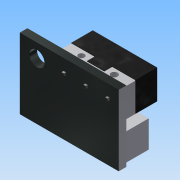
# Autodesk Inventor part: концевик
Saved by Autodesk Inventor 2017 (Build 210142000, 142)
## iProperties
Part Number: концевик
Material: Типовые
Document SubType Name: Modeling
Designer: chucha
Density: 1 g/cm^3
Appearance: Оружейный металл — полированный
Mass: 0.936935 g
Surface Area: 11.9295 cm^2
Volume: 0.936935 cm^3
Author: chucha
Autodesk Inventor part; units mm, degrees
ref_plane "YZ Plane" through (0, 0, 0) normal (1, 0, 0) x (0, 1, 0)
ref_plane "XZ Plane" through (0, 0, 0) normal (0, 1, 0) x (-1, 0, 0)
sketch "Эскиз1" plane through (0, 0, 0) normal (0, 0, 1) x (1, 0, 0)
  line L0 (0, 0) -> (0, 34.3761) construction
  line L1 (0, 0) -> (-29.3608, 0) construction
  circle A0 centre (-10, 0) radius 1.65
  circle A1 centre (-10, 0) radius 3.45
  circle A2 centre (10, 0) radius 1.65
  circle A3 centre (10, 0) radius 3.45
  line L2 (-10, 3.45) -> (10, 3.45)
  line L3 (-6.5, -3.45) -> (-6.5, -9.66)
  line L4 (-6.5, -9.66) -> (6.5, -9.66)
  line L5 (6.5, -9.66) -> (6.5, -3.45)
  line L6 (-10, -3.45) -> (-6.5, -3.45)
  line L7 (6.5, -3.45) -> (10, -3.45)
  line L8 (-4.98, -7.06) -> (4.98, -7.06)
  line L9 (4.98, -7.06) -> (4.98, -14)
  line L10 (4.98, -14) -> (-4.98, -14)
  line L11 (-4.98, -14) -> (-4.98, -7.06)
  line L12 (-6.38, 8.03) -> (6.38, 8.03)
  line L13 (-6.38, 3.7894) -> (-1.7, 3.7894)
  line L14 (-1.7, 3.7894) -> (-1.7, 2.21)
  line L15 (-1.7, 2.21) -> (1.7, 2.21)
  line L16 (1.7, 2.21) -> (1.7, 3.7894)
  line L17 (1.7, 3.7894) -> (6.38, 3.7894)
  line L18 (-6.38, 3.6894) -> (-6.29, 3.6894)
  line L19 (-6.29, 3.6894) -> (-6.29, 3.7894)
  line L20 (6.38, 3.6894) -> (6.29, 3.6894)
  line L21 (6.29, 3.6894) -> (6.29, 3.7894)
  line L22 (-6.38, 1.91) -> (-6.38, 3.6894)
  line L23 (-6.38, 3.7894) -> (-6.38, 8.03)
  line L24 (6.38, 8.03) -> (6.38, 3.7894)
  line L25 (6.38, 3.6894) -> (6.38, 1.91)
  line L26 (-6.38, 1.91) -> (-4.4028, 1.91)
  line L27 (-4.4028, 1.91) -> (-4, 1.43)
  line L28 (6.38, 1.91) -> (4.4028, 1.91)
  line L29 (4.4028, 1.91) -> (4, 1.43)
  line L30 (-2.5, 1.43) -> (-2.0972, 1.91)
  line L31 (-2.0972, 1.91) -> (2.0972, 1.91)
  line L32 (2.0972, 1.91) -> (2.5, 1.43)
  circle A4 centre (-3.25, 2.6493) radius 0.6032
  circle A5 centre (3.25, 2.6493) radius 0.6676
  line L33 (-3.25, 2.6493) -> (-3.25, 0.6364) construction
  line L34 (3.25, 2.6493) -> (3.25, 0.375) construction
  line L35 (4, 1.43) -> (2.5, 1.43)
  line L36 (-2.5, 1.43) -> (-4, 1.43)
  circle A6 centre (10, 0) radius 3.45
  dimension "d0" = 3.3
  dimension "d1" = 6.9
  dimension "d2" = 3.3
  dimension "d3" = 6.9
  dimension "d4" = 20
  dimension "d5" = 26.9
  dimension "d6" = 13.11
  dimension "d7" = 6.21
  dimension "d8" = 13
  dimension "d9" = 2.6
  dimension "d10" = 6.94
  dimension "d11" = 9.96
  dimension "d14" = 4.58
  dimension "d15" = 0.1
  dimension "d16" = 6.38
  dimension "d17" = 6.38
  dimension "d18" = 6.38
  dimension "d19" = 6.38
  dimension "d20" = 6.12
  dimension "d21" = 0.3
  dimension "d22" = 6.6
  dimension "d23" = 130
  dimension "d24" = 3.4
  dimension "d25" = 6.5
  dimension "d26" = 1.5
  constraints: 74 end point, 14 parallel, 10 perpendicular, 7 horizontal, 6 centre point, 5 point on line, 4 collinear, 4 point on circle, 4 vertical, 3 coincident, 3 tangent, 2 symmetric about line, 1 vertical alignment, 9 other
  measures "d0" diameter of A0
  measures "d1" diameter of A1
  measures "d2" diameter of A2
  measures "d3" diameter of A3
  measures "d4" distance of A0.centre A2.centre
  measures "d6" distance between parallel lines of L2 L4
  measures "d7" distance between parallel lines of L4 L6
  measures "d8" distance between parallel lines of L5 L3
  measures "d9" distance between parallel lines of L4 L8
  measures "d10" distance between parallel lines of L10 L8
  measures "d11" distance between parallel lines of L9 L11
  measures "d14" distance between parallel lines of L12 L2
  measures "d15" distance between parallel lines of L18 L13
  measures "d16" distance between parallel lines of L0 L23
  measures "d17" distance between parallel lines of L0 L24
  measures "d18" distance between parallel lines of L0 L22
  measures "d19" distance between parallel lines of L0 L25
  measures "d20" distance between parallel lines of L12 L26
  measures "d21" distance between parallel lines of L31 L15
  measures "d22" distance between parallel lines of L12 L36
  measures "d23" angle of L26 L27
  measures "d24" distance between parallel lines of L16 L14
  measures "d25" distance between parallel lines of L34 L33
  measures "d26" distance of L30.start L27.end
extrude "Выдавливание1" add sketch "Эскиз1" against normal blind 1.55 contours A1 | A1 L2 L22 L26 L27 L36 L30 L31 L32 L35 L29 L28 L25 A3 L7 L5 L4 L9 L8 L11 L3 L6 | L2 L14 L15 L16 L25 L28 L29 L35 L32 L31 L30 L36 L27 L26 L22 | L2 L16 L15 L14 | L11 L8 L9 L4 | A3 | A4 | A5
extrude "Выдавливание2" add sketch "Эскиз1" along normal blind 5.8 contours L14 L13 L23 L12 L24 L17 L16 L2 | L2 L16 L15 L14
extrude "Выдавливание3" add sketch "Эскиз1" along normal blind 5.7 contours L22 L18 L19 L13 L14 L2 | L2 L14 L15 L16 L25 L28 L29 L35 L32 L31 L30 L36 L27 L26 L22 | L16 L17 L21 L20 L25 L2
extrude "Выдавливание4" add sketch "Эскиз1" along normal blind 0.05 contours A1 | A3
extrude "Выдавливание5" add sketch "Эскиз1" along normal blind 5.8 contours L11 L8 L9 L4 | L4 L9 L10 L11
sketch "Эскиз2" plane through (-4.98, -14, 0) normal (0, -1, 0) x (1, 0, 0)
  line L0 (9.96, 0) -> (0, 0) projected
  line L1 (9.96, 0) -> (9.96, 5.8) projected
  line L2 (0, 5.8) -> (9.96, 5.8) projected
  line L3 (0, 0) -> (0, 5.8) projected
  line L4 (4.98, 0) -> (4.98, 10.0399) construction
  line L5 (0, 0) -> (0, 5.8) construction
  line L6 (0, 2.9) -> (8.4494, 2.9) construction
  line L7 (9.41, 0.55) -> (0.55, 0.55)
  line L8 (0.55, 0.55) -> (0.55, 5.25)
  line L9 (0.55, 5.25) -> (9.41, 5.25)
  line L10 (9.41, 5.25) -> (9.41, 0.55)
  line L11 (9.41, 0.55) -> (0.55, 5.25) construction
  line L12 (0.55, 0.55) -> (9.41, 5.25) construction
  line L13 (0, 5.25) -> (9.96, 5.25)
  line L14 (9.96, 5.25) -> (9.96, 4.05)
  line L15 (9.96, 4.05) -> (0, 4.05)
  line L16 (0, 4.05) -> (0, 5.25)
  line L17 (9.96, 5.8) -> (0, 5.8) projected
  line L18 (1.78, 5.25) -> (3.58, 5.25)
  line L19 (3.58, 5.25) -> (3.58, 5.8)
  line L20 (3.58, 5.8) -> (1.78, 5.8)
  line L21 (1.78, 5.8) -> (1.78, 5.25)
  line L22 (6.38, 5.25) -> (8.18, 5.25)
  line L23 (8.18, 5.25) -> (8.18, 5.8)
  line L24 (8.18, 5.8) -> (6.38, 5.8)
  line L25 (6.38, 5.8) -> (6.38, 5.25)
  line L26 (-3.9038, 3.4362) -> (13.6375, 3.4362) construction
  line L27 (5.23, 3.6862) -> (4.73, 3.6862)
  line L28 (4.73, 3.6862) -> (4.73, 3.1862)
  line L29 (4.73, 3.1862) -> (5.23, 3.1862)
  line L30 (5.23, 3.1862) -> (5.23, 3.6862)
  line L31 (5.23, 3.6862) -> (4.73, 3.1862) construction
  line L32 (4.73, 3.6862) -> (5.23, 3.1862) construction
  line L33 (2.73, 3.6862) -> (2.23, 3.6862)
  line L34 (2.23, 3.6862) -> (2.23, 3.1862)
  line L35 (2.23, 3.1862) -> (2.73, 3.1862)
  line L36 (2.73, 3.1862) -> (2.73, 3.6862)
  line L37 (2.73, 3.6862) -> (2.23, 3.1862) construction
  line L38 (2.23, 3.6862) -> (2.73, 3.1862) construction
  line L39 (7.23, 3.6862) -> (7.73, 3.6862)
  line L40 (7.73, 3.6862) -> (7.73, 3.1862)
  line L41 (7.73, 3.1862) -> (7.23, 3.1862)
  line L42 (7.23, 3.1862) -> (7.23, 3.6862)
  line L43 (7.23, 3.6862) -> (7.73, 3.1862) construction
  line L44 (7.73, 3.6862) -> (7.23, 3.1862) construction
  line L45 (0.5772, 0) -> (0.5772, 5.7) projected
  line L46 (0, 5.25) -> (0.5772, 5.25)
  line L47 (0.5772, 5.25) -> (0.5772, 4.05)
  line L48 (0.5772, 4.05) -> (0, 4.05)
  line L49 (0, 4.05) -> (0, 5.25)
  line L50 (9.96, 5.25) -> (9.41, 5.25)
  line L51 (9.41, 5.25) -> (9.41, 4.05)
  line L52 (9.41, 4.05) -> (9.96, 4.05)
  line L53 (9.96, 4.05) -> (9.96, 5.25)
  line L54 (8.18, 5.25) -> (6.38, 5.25)
  line L55 (6.38, 5.25) -> (6.38, 5.8)
  line L56 (6.38, 5.8) -> (8.18, 5.8)
  line L57 (8.18, 5.8) -> (8.18, 5.25)
  line L58 (3.58, 5.25) -> (1.78, 5.25)
  line L59 (1.78, 5.25) -> (1.78, 5.8)
  line L60 (1.78, 5.8) -> (3.58, 5.8)
  line L61 (3.58, 5.8) -> (3.58, 5.25)
  point P0 (4.98, 2.9)
  point P1 (4.98, 3.4362)
  point P2 (2.48, 3.4362)
  point P3 (7.48, 3.4362)
  dimension "d37" = 0.55
  dimension "d38" = 0.55
  dimension "d39" = 1.2
  dimension "d40" = 1.8
  dimension "d41" = 1.8
  dimension "d42" = 2.8
  dimension "d43" = 0.5
  dimension "d44" = 0.5
  dimension "d45" = 0.5
  dimension "d46" = 0.5
  dimension "d47" = 5
  constraints: 110 end point, 22 parallel, 18 point on line, 13 horizontal, 11 perpendicular, 9 midpoint, 1 collinear, 1 symmetric about line, 1 vertical, 1 other
  measures "d37" distance between parallel lines of L2 L9
  measures "d38" distance between parallel lines of L3 L8
  measures "d39" distance between parallel lines of L15 L13
  measures "d40" distance between parallel lines of L23 L25
  measures "d41" distance between parallel lines of L21 L19
  measures "d42" distance between parallel lines of L25 L19
  measures "d43" distance of L29.end L28.end
  measures "d44" distance of L28.end L27.end
  measures "d45" distance of L35.end L34.end
  measures "d46" distance of L40.end L41.end
  measures "d47" distance of point (2.48, 3.436) point (7.48, 3.436)
extrude "Выдавливание6" cut sketch "Эскиз2" against normal blind 5.3 contours L45 L15 L10 L7 | L7 L8 L15 L45 | L15 L45 L9 L10 | L15 L8 L9 L45
extrude "Выдавливание7" cut sketch "Эскиз2" against normal blind 3.2 contours L15 L10 L13 L1 | L3 L13 L8 L15 | L15 L8 L9 L45 | L23 L9 L25 L2 | L21 L2 L19 L9
sketch "Эскиз3" plane through (0, 0, 0) normal (1, 0, 0) x (0, 1, 0)
  line L0 (2.5743, 3.55) -> (-0.5, 3.55)
  line L1 (0, 3.05) -> (2.5743, 3.05)
  line L2 (2.5743, 3.05) -> (2.5743, 3.55)
  line L3 (0, 3.05) -> (0, 0)
  line L4 (0, 0) -> (-0.5, 0)
  line L5 (-0.5, 0) -> (-0.5, 3.55)
  line L6 (-7.06, 0) -> (-7.06, 5.8) projected
  line L7 (-3.45, 0) -> (-9.66, 0) projected
  line L8 (-7.06, 3.686) -> (-6.36, 3.686)
  line L9 (-6.36, 3.686) -> (-6.36, 0)
  line L10 (-6.36, 0) -> (-7.06, 0)
  line L11 (-7.06, 0) -> (-7.06, 3.686)
  line L12 (-7.06, 3.186) -> (-6.86, 3.186)
  line L13 (-6.86, 3.186) -> (-6.86, 0)
  line L14 (-6.86, 0) -> (-7.06, 0)
  line L15 (-7.06, 0) -> (-7.06, 3.186)
  line L16 (1.91, 0) -> (1.91, 5.7) projected
  line L17 (3.45, 0.05) -> (-3.45, 0.05) projected
  dimension "d52" = 3.686
  dimension "d53" = 0.5
  dimension "d54" = 0.5
  dimension "d55" = 0.2
  dimension "d56" = 0.5
  dimension "d57" = 0.5
  dimension "d58" = 2.41
  dimension "d59" = 3.5
  constraints: 28 end point, 6 parallel, 4 point on line, 3 horizontal, 2 perpendicular
  measures "d52" distance between parallel lines of L7 L8
  measures "d53" distance between parallel lines of L8 L12
  measures "d54" distance between parallel lines of L9 L13
  measures "d55" distance between parallel lines of L6 L13
  measures "d56" distance between parallel lines of L5 L3
  measures "d57" distance between parallel lines of L0 L1
  measures "d58" distance between parallel lines of L16 L5
  measures "d59" distance between parallel lines of L17 L0
extrude "Выдавливание9" add sketch "Эскиз3" along normal mid plane 0.5 contours L2 L1 L16 L0 | L16 L1 L3 L17 L5 L0 | L17 L3 L4 L5
pattern_linear "Прямоуг.массив1" count 3 spacing 4.32 along (1, 0, 0) of "Выдавливание9" first direction both ways yes
extrude "Выдавливание10" add sketch "Эскиз3" along normal mid plane 0.5 contours L6 L8 L9 L7 L13 L12
pattern_linear "Прямоуг.массив2" count 3 spacing 1.9 along (1, 0, 0) of "Выдавливание10" first direction both ways yes
sketch "Эскиз4" plane through (0, 0, -1.55) normal (0, 0, -1) x (-1, 0, 0)
  line L0 (-1.65, -6.86) -> (-1.65, -6.36) projected
  line L1 (-1.65, -6.36) -> (-2.15, -6.36) projected
  line L2 (-2.15, -6.36) -> (-2.15, -6.86) projected
  line L3 (-2.15, -6.86) -> (-1.65, -6.86) projected
  line L4 (2.15, -6.86) -> (2.15, -6.36) projected
  line L5 (2.15, -6.36) -> (1.65, -6.36) projected
  line L6 (1.65, -6.36) -> (1.65, -6.86) projected
  line L7 (1.65, -6.86) -> (2.15, -6.86) projected
  line L8 (0.25, -6.86) -> (0.25, -6.36) projected
  line L9 (0.25, -6.36) -> (-0.25, -6.36) projected
  line L10 (-0.25, -6.36) -> (-0.25, -6.86) projected
  line L11 (-0.25, -6.86) -> (0.25, -6.86) projected
  line L12 (-4.07, -0.5) -> (-4.07, 0) projected
  line L13 (-4.07, 0) -> (-4.57, 0) projected
  line L14 (-4.57, 0) -> (-4.57, -0.5) projected
  line L15 (-4.57, -0.5) -> (-4.07, -0.5) projected
  line L16 (4.57, -0.5) -> (4.57, 0) projected
  line L17 (4.57, 0) -> (4.07, 0) projected
  line L18 (4.07, 0) -> (4.07, -0.5) projected
  line L19 (4.07, -0.5) -> (4.57, -0.5) projected
  line L20 (0.25, -0.5) -> (0.25, 0) projected
  line L21 (0.25, 0) -> (-0.25, 0) projected
  line L22 (-0.25, 0) -> (-0.25, -0.5) projected
  line L23 (-0.25, -0.5) -> (0.25, -0.5) projected
  line L24 (-4.98, -7.06) -> (-4.98, -9.66) projected
  line L25 (-4.98, -9.66) -> (-6.5, -9.66) projected
  line L26 (-6.5, -9.66) -> (-6.5, -3.45) projected
  line L27 (-6.5, -3.45) -> (-10, -3.45) projected
  arc A0 (-10, -3.45) -> (-10, 3.45) centre (-10, 0) ccw projected
  line L28 (-10, 3.45) -> (-6.38, 3.45) projected
  line L29 (-6.38, 3.45) -> (-6.38, 1.91) projected
  line L30 (-6.38, 1.91) -> (-4.4028, 1.91) projected
  line L31 (-4.4028, 1.91) -> (-4, 1.43) projected
  line L32 (-4, 1.43) -> (-2.5, 1.43) projected
  line L33 (-2.5, 1.43) -> (-2.0972, 1.91) projected
  line L34 (-2.0972, 1.91) -> (2.0972, 1.91) projected
  line L35 (2.0972, 1.91) -> (2.5, 1.43) projected
  line L36 (2.5, 1.43) -> (4, 1.43) projected
  line L37 (4, 1.43) -> (4.4028, 1.91) projected
  line L38 (4.4028, 1.91) -> (6.38, 1.91) projected
  line L39 (6.38, 1.91) -> (6.38, 3.45) projected
  line L40 (6.38, 3.45) -> (10, 3.45) projected
  arc A1 (10, 3.45) -> (10, -3.45) centre (10, 0) ccw projected
  line L41 (10, -3.45) -> (6.5, -3.45) projected
  line L42 (6.5, -3.45) -> (6.5, -9.66) projected
  line L43 (6.5, -9.66) -> (4.98, -9.66) projected
  line L44 (4.98, -9.66) -> (4.98, -7.06) projected
  line L45 (4.98, -7.06) -> (-4.98, -7.06) projected
  point P0 (0, 0)
extrude "Выдавливание11" add sketch "Эскиз4" along normal blind 1.35 contours L3 L2 L1 L0 | L7 L6 L5 L4 | L11 L10 L9 L8 | L15 L14 L13 L12 | L19 L18 L17 L16 | L23 L22 L21 L20
fillet "Сопряжение1" radius 1.1 12 edges at (-1.9, -6.36, -1.55) (0, -6.36, -1.55) (1.9, -6.36, -1.55) (1.9, -6.86, -1.55) (0, -6.86, -1.55) (-1.9, -6.86, -1.55) (-4.32, -0.5, -1.55) (0, -0.5, -1.55) (4.32, -0.5, -1.55) (4.32, 0, -1.55) (0, 0, -1.55) (-4.32, 0, -1.55)
fillet "Сопряжение2" radius 0.6 12 edges at (-4.07, -0.25, -1.55) (0.25, -0.25, -1.55) (4.57, -0.25, -1.55) (2.15, -6.61, -1.55) (0.25, -6.61, -1.55) (-1.65, -6.61, -1.55) (1.65, -6.61, -1.55) (-0.25, -6.61, -1.55) (-2.15, -6.61, -1.55) (-4.57, -0.25, -1.55) (-0.25, -0.25, -1.55) (4.07, -0.25, -1.55)
sketch "Эскиз5" plane through (0, 0, -1.55) normal (0, 0, -1) x (-1, 0, 0)
  arc A0 (-10, -3.45) -> (-10, 3.45) centre (-10, 0) ccw projected
  arc A1 (10, 3.45) -> (10, -3.45) centre (10, 0) ccw projected
  circle A2 centre (-10, 0) radius 3.45
  line L0 (10, 3.45) -> (-10, 3.45) projected
  circle A3 centre (10, 0) radius 3.45
  point P0 (0, 0)
  constraints: 2 coincident, 2 vertical alignment, 4 other
extrude "Выдавливание12" cut sketch "Эскиз5" against normal blind 0.01
sketch "Эскиз6" plane through (0, 0, 0) normal (0, 0, 1) x (1, 0, 0)
  line L0 (-6.5, -3.45) -> (-6.5, -9.66) projected
  line L1 (6.5, -9.66) -> (6.5, -3.45) projected
  line L2 (-6.5, -3.45) -> (6.5, -3.45)
  line L3 (6.5, -3.45) -> (6.5, -4.7506)
  line L4 (6.5, -4.7506) -> (-6.5, -4.7506)
  line L5 (-6.5, -4.7506) -> (-6.5, -3.45)
  line L6 (-6.3, -3.65) -> (-3.3, -3.65)
  line L7 (-3.3, -3.65) -> (-3.3, -4.5506)
  line L8 (-3.3, -4.5506) -> (-6.3, -4.5506)
  line L9 (-6.3, -4.5506) -> (-6.3, -3.65)
  line L10 (3.3, -3.65) -> (6.3, -3.65)
  line L11 (6.3, -3.65) -> (6.3, -4.5506)
  line L12 (6.3, -4.5506) -> (3.3, -4.5506)
  line L13 (3.3, -4.5506) -> (3.3, -3.65)
  line L14 (0, 0) -> (0, -22.5011) construction
  line L15 (-3.1, -3.65) -> (-0.1, -3.65)
  line L16 (-0.1, -3.65) -> (-0.1, -4.5506)
  line L17 (-0.1, -4.5506) -> (-3.1, -4.5506)
  line L18 (-3.1, -4.5506) -> (-3.1, -3.65)
  line L19 (0.1, -3.65) -> (3.1, -3.65)
  line L20 (3.1, -3.65) -> (3.1, -4.5506)
  line L21 (3.1, -4.5506) -> (0.1, -4.5506)
  line L22 (0.1, -4.5506) -> (0.1, -3.65)
  line L23 (-6.1, -3.85) -> (-3.5, -3.85)
  line L24 (-3.5, -3.85) -> (-3.5, -4.3506)
  line L25 (-3.5, -4.3506) -> (-6.1, -4.3506)
  line L26 (-6.1, -4.3506) -> (-6.1, -3.85)
  line L27 (-2.9, -3.85) -> (-0.3, -3.85)
  line L28 (-0.3, -3.85) -> (-0.3, -4.3506)
  line L29 (-0.3, -4.3506) -> (-2.9, -4.3506)
  line L30 (-2.9, -4.3506) -> (-2.9, -3.85)
  line L31 (0.3, -3.85) -> (2.9, -3.85)
  line L32 (2.9, -3.85) -> (2.9, -4.3506)
  line L33 (2.9, -4.3506) -> (0.3, -4.3506)
  line L34 (0.3, -4.3506) -> (0.3, -3.85)
  line L35 (3.5, -3.85) -> (6.1, -3.85)
  line L36 (6.1, -3.85) -> (6.1, -4.3506)
  line L37 (6.1, -4.3506) -> (3.5, -4.3506)
  line L38 (3.5, -4.3506) -> (3.5, -3.85)
  line L39 (-5.6, -3.85) -> (-4, -3.85)
  line L40 (-4, -3.85) -> (-4, -4.3506)
  line L41 (-4, -4.3506) -> (-5.6, -4.3506)
  line L42 (-5.6, -4.3506) -> (-5.6, -3.85)
  line L43 (-2.4, -3.85) -> (-0.8, -3.85)
  line L44 (-0.8, -3.85) -> (-0.8, -4.3506)
  line L45 (-0.8, -4.3506) -> (-2.4, -4.3506)
  line L46 (-2.4, -4.3506) -> (-2.4, -3.85)
  line L47 (0.8, -3.85) -> (2.4, -3.85)
  line L48 (2.4, -3.85) -> (2.4, -4.3506)
  line L49 (2.4, -4.3506) -> (0.8, -4.3506)
  line L50 (0.8, -4.3506) -> (0.8, -3.85)
  line L51 (4, -3.85) -> (5.6, -3.85)
  line L52 (5.6, -3.85) -> (5.6, -4.3506)
  line L53 (5.6, -4.3506) -> (4, -4.3506)
  line L54 (4, -4.3506) -> (4, -3.85)
  dimension "d78" = 0.2
  dimension "d79" = 0.2
  dimension "d80" = 0.2
  dimension "d81" = 0.2
  dimension "d82" = 0.2
  dimension "d83" = 0.2
  dimension "d84" = 0.2
  dimension "d85" = 3
  dimension "d86" = 3
  dimension "d87" = 0.2
  dimension "d88" = 0.2
  dimension "d89" = 0.2
  dimension "d90" = 0.2
  dimension "d91" = 0.2
  dimension "d92" = 0.2
  dimension "d93" = 2.6
  dimension "d94" = 0.5
  dimension "d95" = 0.5
  dimension "d96" = 0.5
  dimension "d97" = 0.5
  constraints: 106 end point, 26 parallel, 19 point on line, 13 horizontal, 13 perpendicular, 2 collinear, 1 vertical, 11 other
  measures "d78" distance between parallel lines of L2 L6
  measures "d79" distance between parallel lines of L0 L9
  measures "d80" distance between parallel lines of L4 L8
  measures "d81" distance between parallel lines of L18 L7
  measures "d82" distance between parallel lines of L13 L20
  measures "d83" distance between parallel lines of L22 L16
  measures "d84" distance between parallel lines of L4 L17
  measures "d85" distance between parallel lines of L7 L9
  measures "d86" distance between parallel lines of L16 L18
  measures "d87" distance between parallel lines of L9 L26
  measures "d88" distance between parallel lines of L7 L24
  measures "d89" distance between parallel lines of L30 L18
  measures "d90" distance between parallel lines of L16 L28
  measures "d91" distance between parallel lines of L17 L29
  measures "d92" distance between parallel lines of L19 L31
  measures "d93" distance between parallel lines of L36 L38
  measures "d94" distance between parallel lines of L36 L52
  measures "d95" distance between parallel lines of L38 L54
  measures "d96" distance between parallel lines of L32 L48
  measures "d97" distance between parallel lines of L50 L34
extrude "Выдавливание13" add sketch "Эскиз6" along normal blind 0.01 contours L2 L1 L4 L0
extrude "Выдавливание14" add sketch "Эскиз6" along normal blind 0.8 contours L23 L40 L25 L42 | L27 L44 L29 L46 | L31 L48 L33 L50 | L35 L52 L37 L54
extrude "Выдавливание15" add sketch "Эскиз6" along normal blind 0.4 contours L23 L42 L25 L26 | L23 L40 L25 L42 | L23 L24 L25 L40 | L27 L46 L29 L30 | L27 L44 L29 L46 | L27 L28 L29 L44 | L31 L50 L33 L34 | L31 L48 L33 L50 | L31 L32 L33 L48 | L35 L54 L37 L38 | L35 L52 L37 L54 | L35 L36 L37 L52
fillet "Сопряжение3" radius 0.3 8 edges at (-5.6, -4.1003, 0.4) (-2.4, -4.1003, 0.4) (0.8, -4.1003, 0.4) (4, -4.1003, 0.4) (5.6, -4.1003, 0.4) (2.4, -4.1003, 0.4) (-0.8, -4.1003, 0.4) (-4, -4.1003, 0.4)
ref_plane "РабПлоскость1" through (0, 0, 2.9) normal (0, 0, 1) x (1, 0, 0)
sketch "Эскиз9" plane through (-6.38, 8.03, 0) normal (0, 1, 0) x (1, 0, 0)
  line L0 (4.55, -1.3703) -> (3.6, -1.3703)
  line L1 (3.6, -1.3703) -> (3.6, -4.3825)
  line L2 (3.6, -4.3825) -> (4.55, -4.3825)
  line L3 (4.55, -4.3825) -> (4.55, -1.3703)
  line L4 (0, 0) -> (0, -5.8) projected
  point P0 (6.38, 0)
  dimension "d119" = 4.55
  dimension "d120" = 0.95
  constraints: 8 end point, 2 parallel, 1 horizontal, 1 perpendicular
  measures "d119" distance between parallel lines of L4 L3
  measures "d120" distance between parallel lines of L1 L3
extrude "Выдавливание18" add sketch "Эскиз9" along normal blind 1
sketch "Эскиз10" plane through (0, 0, 0) normal (0, 0, 1) x (1, 0, 0)
  line L0 (-16.5801, -25.0407) -> (19.4758, -25.0407)
  line L1 (19.4758, -25.0407) -> (19.4758, 14.3607)
  line L2 (19.4758, 14.3607) -> (-16.5801, 14.3607)
  line L3 (-16.5801, 14.3607) -> (-16.5801, -25.0407)
  point P0 (0, 0)
  constraints: 8 end point, 2 parallel, 1 horizontal, 1 perpendicular
extrude "Выдавливание19" cut sketch "Эскиз10" against normal blind 10
sketch "Эскиз11" plane through (0, 0, 5.8) normal (0, 0, 1) x (1, 0, 0)
  circle A0 centre (-10, 0) radius 1.65 projected
  circle A1 centre (-10, 0) radius 3.45 projected
  circle A2 centre (10, 0) radius 1.65 projected
  circle A3 centre (10, 0) radius 3.45 projected
  circle A4 centre (10, 0) radius 1.65 projected
  line L0 (-10.5534, -19.0482) -> (10, -19.0482)
  line L1 (10, -19.0482) -> (10, 0)
  line L2 (10, 0) -> (-10.5534, 0)
  line L3 (-10.5534, 0) -> (-10.5534, -19.0482)
  point P0 (0, 0)
  constraints: 8 end point, 2 parallel, 1 horizontal, 1 perpendicular
extrude "Выдавливание20" cut sketch "Эскиз11" against normal blind 10
sketch "Эскиз12" plane through (-6.38, 1.91, 5.7) normal (0, -1, 0) x (1, 0, 0)
  line L0 (8.08, 0.1) -> (12.76, 0.1) projected
  line L1 (12.76, 0.1) -> (-6.84, 0.1)
  line L2 (-6.84, 0.1) -> (-6.84, -13.9)
  line L3 (-6.84, -13.9) -> (12.76, -13.9)
  line L4 (12.76, -13.9) -> (12.76, 0.1)
  circle A0 centre (-3.84, -2.9) radius 1.5
  circle A1 centre (10.16, -10.9) radius 1.5
  point P0 (6.38, -5.7)
  dimension "d127" = 14
  dimension "d128" = 19.6
  dimension "d129" = 3
  dimension "d141" = 3
  dimension "d144" = 14
  dimension "d145" = 8
  dimension "d146" = 3
  dimension "d147" = 2.6
  constraints: 8 end point, 2 centre point, 2 parallel, 1 horizontal, 1 perpendicular
  measures "d127" distance between parallel lines of L1 L3
  measures "d128" distance between parallel lines of L4 L2
  measures "d129" diameter of A0
  measures "d141" diameter of A1
  measures "d144" horizontal distance of A1.centre A0.centre
  measures "d145" vertical distance of A0.centre A1.centre
  measures "d146" distance from line of L1 A0.centre
  measures "d147" distance from line of L4 A1.centre
extrude "Выдавливание21" add sketch "Эскиз12" along normal blind 1.5 contours L0 L4 L3 L2 L1 | A1
sketch "Эскиз13" plane through (-6.38, 1.91, 5.7) normal (0, 1, 0) x (1, 0, 0)
  line L0 (2.2889, 13.2364) -> (2.2889, 8.3357)
  line L1 (-5.7194, 13.2364) -> (2.2889, 13.2364)
  line L2 (2.2889, 13.2364) -> (2.2889, 8.3357)
  line L3 (2.2889, 8.3357) -> (-5.7194, 8.3357)
  line L4 (-5.7194, 8.3357) -> (-5.7194, 13.2364)
  point P0 (6.38, 5.7)
  constraints: 10 end point, 2 parallel, 1 horizontal, 1 perpendicular
extrude "Выдавливание22" add sketch "Эскиз13" along normal blind 5
sketch "Эскиз14" plane through (-4.0911, 1.91, -7.5364) normal (0, 0, -1) x (-1, 0, 0)
  line L0 (7.4155, 4.3491) -> (0.812, 4.3491)
  line L1 (0.812, 4.3491) -> (0.812, 0.6352)
  line L2 (0.812, 0.6352) -> (7.4155, 0.6352)
  line L3 (7.4155, 0.6352) -> (7.4155, 4.3491)
  line L4 (6.38, 2.6869) -> (5.9904, 2.6869)
  line L5 (5.9904, 2.6869) -> (5.9904, 2.1156)
  line L6 (5.9904, 2.1156) -> (6.38, 2.1156)
  line L7 (6.38, 2.1156) -> (6.38, 2.6869)
  line L8 (4.7698, 2.6869) -> (4.1984, 2.6869)
  line L9 (4.1984, 2.6869) -> (4.1984, 2.1156)
  line L10 (4.1984, 2.1156) -> (4.7698, 2.1156)
  line L11 (4.7698, 2.1156) -> (4.7698, 2.6869)
  line L12 (3.1336, 2.6869) -> (2.5622, 2.6869)
  line L13 (2.5622, 2.6869) -> (2.5622, 2.1156)
  line L14 (2.5622, 2.1156) -> (3.1336, 2.1156)
  line L15 (3.1336, 2.1156) -> (3.1336, 2.6869)
  point P0 (-4.0911, -1.91)
  constraints: 32 end point, 8 parallel, 4 horizontal, 4 perpendicular, 4 point on line
extrude "Выдавливание23" cut sketch "Эскиз14" against normal blind 4
sketch "Эскиз16" plane through (-6.38, 1.91, 5.7) normal (0, 1, 0) x (1, 0, 0)
  line L0 (-5.7194, 8.3357) -> (2.2889, 8.3357) projected
  line L1 (-3.5285, 6.8998) -> (-2.9759, 6.8998)
  line L2 (-2.9759, 6.8998) -> (-2.9759, 8.3357)
  line L3 (-2.9759, 8.3357) -> (-3.5285, 8.3357)
  line L4 (-3.5285, 8.3357) -> (-3.5285, 6.8998)
  line L5 (-2.3178, 6.8998) -> (-1.7152, 6.8998)
  line L6 (-1.7152, 6.8998) -> (-1.7152, 8.3357)
  line L7 (-1.7152, 8.3357) -> (-2.3178, 8.3357)
  line L8 (-2.3178, 8.3357) -> (-2.3178, 6.8998)
  line L9 (-1.0271, 6.8998) -> (-0.4589, 6.8998)
  line L10 (-0.4589, 6.8998) -> (-0.4589, 8.3357)
  line L11 (-0.4589, 8.3357) -> (-1.0271, 8.3357)
  line L12 (-1.0271, 8.3357) -> (-1.0271, 6.8998)
  point P0 (6.38, 5.7)
  constraints: 24 end point, 6 parallel, 4 point on line, 3 horizontal, 3 perpendicular, 1 midpoint
extrude "Выдавливание24" add sketch "Эскиз16" along normal blind 3
fillet "Сопряжение4" radius 1 3 edges at (-9.6322, 4.91, -1.1998) (-8.3965, 4.91, -1.1998) (-7.123, 4.91, -1.1998)
sketch "Эскиз17" plane through (-6.38, 6.91, 5.7) normal (0, 1, 0) x (1, 0, 0)
  line L0 (-4.8044, 11.3398) -> (-4.0958, 11.3398)
  line L1 (-4.0958, 11.3398) -> (-4.0958, 13.5942)
  line L2 (-4.0958, 13.5942) -> (-4.8044, 13.5942)
  line L3 (-4.8044, 13.5942) -> (-4.8044, 11.3398)
  line L4 (0.4774, 11.3398) -> (1.2181, 11.3398)
  line L5 (1.2181, 11.3398) -> (1.2181, 14.0773)
  line L6 (1.2181, 14.0773) -> (0.4774, 14.0773)
  line L7 (0.4774, 14.0773) -> (0.4774, 11.3398)
  point P0 (6.38, 5.7)
  constraints: 16 end point, 4 parallel, 2 horizontal, 2 perpendicular, 1 point on line
extrude "Выдавливание25" cut sketch "Эскиз17" against normal blind 3
extrude "Выдавливание26" cut sketch "Эскиз12" along normal blind 3 contours A1
